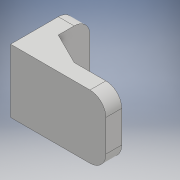
# Autodesk Inventor part: 33
Saved by Autodesk Inventor 2017 (Build 210142000, 142)
## iProperties
Part Number: 33
Material: 一般
Document SubType Name: Modeling
Designer: Brian
Density: 1 g/cm^3
Appearance: 預設
Author: Brian
Autodesk Inventor part; units mm, degrees
ref_plane "YZ Plane" through (0, 0, 0) normal (1, 0, 0) x (0, 1, 0)
ref_plane "XZ Plane" through (0, 0, 0) normal (0, 1, 0) x (-1, 0, 0)
ref_plane "XY Plane" through (0, 0, 0) normal (0, 0, 1) x (1, 0, 0)
sketch "草圖1" plane through (0, 0, 0) normal (0, 0, 1) x (1, 0, 0)
  line L0 (0, 0) -> (60, 0)
  line L1 (60, 0) -> (60, 10)
  line L2 (60, 10) -> (0, 10)
  line L3 (0, 10) -> (0, 0)
  line L4 (0, 10) -> (10, 10)
  line L5 (10, 10) -> (10, 40)
  line L6 (10, 40) -> (0, 40)
  line L7 (0, 40) -> (0, 10)
  dimension "d0" = 10
  dimension "d1" = 30
  dimension "d2" = 60
  dimension "d3" = 10
  constraints: 16 end point, 4 parallel, 2 horizontal, 2 perpendicular
  measures "d0" distance of L2.end L0.start
  measures "d1" distance of L6.end L2.end
  measures "d2" distance of L0.start L0.end
  measures "d3" distance between parallel lines of L7 L5
extrude "擠出1" add sketch "草圖1" against normal blind 40
chamfer "倒角1" distance 10 distance2 20 1 edges at (10, 10, -20) measured on face at (10, 20, -13.3333)
fillet "圓角1" radius 10 4 edges at (5, 40, 0) (5, 40, -40) (60, 5, 0) (60, 5, -40)
